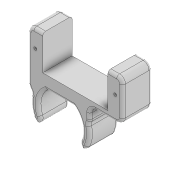
# Autodesk Inventor part: frame_3
Saved by Autodesk Inventor 2022 (Build 260153000, 153)
## iProperties
Created: 2023-05-17
Part Number: frame_3
Material: 일반
Document SubType Name: Modeling
Designer: HCI-TECH_KDK
Density: 1 g/cm^3
Appearance: 기본값
Author: HCI-TECH_KDK
Autodesk Inventor part; units mm, degrees
ref_plane "YZ Plane" through (0, 0, 0) normal (1, 0, 0) x (0, 1, 0)
ref_plane "XZ Plane" through (0, 0, 0) normal (0, 1, 0) x (-1, 0, 0)
ref_plane "XY Plane" through (0, 0, 0) normal (0, 0, 1) x (1, 0, 0)
sketch "스케치1" plane through (0, 0, 0) normal (0, 0, 1) x (1, 0, 0)
  line L0 (0, 0) -> (22.2, 0)
  line L1 (22.2, 0) -> (22.2, 11.8)
  line L2 (22.2, 11.8) -> (0, 11.8)
  line L3 (0, 11.8) -> (0, 0)
  circle A0 centre (6, 5.9) radius 1.877933
  line L4 (-9, 5.9) -> (21, 5.9)
  line L5 (21, 5.9) -> (21, -16.1)
  line L6 (21, -16.1) -> (-9, -16.1)
  line L7 (-9, -16.1) -> (-9, 5.9)
  line L8 (-24.543137, -4.6) -> (59.052201, -4.6) construction
  line L9 (-2, 5.9) -> (14, 5.9) construction
  line L10 (14, 5.9) -> (14, -16.1) construction
  line L11 (14, -16.1) -> (-2, -16.1) construction
  line L12 (-2, -16.1) -> (-2, 5.9) construction
  line L13 (-5, 11.8) -> (27.2, 11.8)
  line L14 (27.2, 11.8) -> (27.2, 0)
  line L15 (27.2, 0) -> (-5, 0)
  line L16 (-5, 0) -> (-5, 11.8)
  point P0 (6, 5.9)
  point P1 (6, 5.9)
  point P2 (0, 5.9)
  point P3 (11.1, 11.8)
  point P4 (11.1, 11.8)
  dimension "d0" = 22.2
  dimension "d1" = 11.8
  dimension "d2" = 6
  dimension "d3" = 22
  dimension "d4" = 30
  dimension "d5" = 11.5
  dimension "d6" = 16
  dimension "d10" = 32.2
  constraints: 34 end point, 8 parallel, 5 horizontal, 5 midpoint, 4 coincident, 4 perpendicular, 2 point on line, 1 centre point, 1 horizontal alignment
  measures "d0" distance of L1.end L2.end
  measures "d1" distance of L0.end L1.end
  measures "d2" distance from line of L3 A0.centre
  measures "d3" distance of L4.end L5.end
  measures "d4" distance of L5.end L6.end
  measures "d5" distance between parallel lines of L6 L8
  measures "d6" distance between parallel lines of L12 L10
  measures "d10" distance of L13.start L13.end
sketch "스케치2" plane through (0, 0, 0) normal (0, 0, 1) x (1, 0, 0)
  line L0 (-24.543137, -4.6) -> (59.052201, -4.6) construction
  line L1 (-2, -16.1) -> (-2, 5.9) construction
  line L2 (14, 5.9) -> (14, -16.1) construction
  line L3 (21, -16.1) -> (-9, -16.1)
  line L4 (-2, -4.6) -> (14, -4.6)
  line L5 (14, -4.6) -> (14, -16.1)
  line L6 (14, -16.1) -> (-2, -16.1)
  line L7 (-2, -16.1) -> (-2, -4.6)
  line L8 (-4, -18.1) -> (16, -18.1)
  line L9 (16, -18.1) -> (16, -2.6)
  line L10 (16, -2.6) -> (-4, -2.6)
  line L11 (-4, -2.6) -> (-4, -18.1)
  point P0 (0, 0)
  point P1 (-2, -16.1)
  dimension "d7" = 2
  dimension "d42" = 11.5
  dimension "d43" = 16
  constraints: 16 end point, 4 parallel, 2 perpendicular, 2 point on line, 1 horizontal, 3 other
  measures "d7" distance between parallel lines of L6 L8
  measures "d42" distance of L6.end L4.start
  measures "d43" distance between parallel lines of L2 L1
sketch "스케치2 outline for 돌출1" plane through (0, 0, 0) normal (0, 0, 1) x (1, 0, 0)
  line L0 (-4, -2.6) -> (-4, -18.1)
  line L1 (16, -2.6) -> (-4, -2.6)
  line L2 (-4, -18.1) -> (16, -18.1)
  line L3 (16, -18.1) -> (16, -2.6)
  line L4 (-2, -16.1) -> (-2, -4.6)
  line L5 (14, -16.1) -> (-2, -16.1)
  line L6 (14, -4.6) -> (14, -16.1)
  line L7 (-2, -4.6) -> (14, -4.6)
extrude "돌출1" add sketch "스케치2 outline for 돌출1" against normal blind 10
sketch "스케치3" plane through (0, 0, 0) normal (0, 0, 1) x (1, 0, 0)
  line L0 (0, 11.8) -> (0, 0)
  line L1 (-5, 11.8) -> (27.2, 11.8)
  line L2 (-5, 0) -> (-5, 11.8)
  line L3 (27.2, 0) -> (-5, 0)
  line L4 (27.2, 11.8) -> (27.2, 0)
  line L5 (22.2, 0) -> (22.2, 11.8)
  line L6 (27.2, 11.8) -> (22.2, 11.8)
  line L7 (27.2, 0) -> (27.2, -6.593642)
  line L8 (27.2, -6.593642) -> (16, -6.593642)
  line L9 (16, -2.6) -> (16, -18.1)
  line L10 (-9, -16.1) -> (-9, 5.9)
  line L11 (-4, -18.1) -> (-4, -2.6)
  line L12 (-4, -6.593642) -> (-9, -6.593642)
  line L13 (-9, 5.9) -> (0, 5.9)
  line L14 (21, 5.9) -> (21, -16.1)
  line L15 (0, 0) -> (22.2, 0)
  line L16 (16, -2.6) -> (-4, -2.6)
  line L17 (16, -18.1) -> (16, -2.6)
  point P0 (-5, 5.9)
  constraints: 10 end point, 3 point on line, 2 perpendicular, 1 collinear, 1 midpoint, 1 vertical
sketch "스케치3 outline for 돌출2" plane through (0, 0, 0) normal (0, 0, 1) x (1, 0, 0)
  line L0 (-4, -2.6) -> (16, -2.6)
  line L1 (-4, -6.593642) -> (-4, -2.6)
  line L2 (-9, -6.593642) -> (-4, -6.593642)
  line L3 (-9, 5.9) -> (-9, -6.593642)
  line L4 (-5, 5.9) -> (-9, 5.9)
  line L5 (-5, 11.8) -> (-5, 5.9)
  line L6 (0, 11.8) -> (-5, 11.8)
  line L7 (0, 0) -> (0, 11.8)
  line L8 (22.2, 0) -> (0, 0)
  line L9 (22.2, 11.8) -> (22.2, 0)
  line L10 (27.2, 11.8) -> (22.2, 11.8)
  line L11 (27.2, 0) -> (27.2, 11.8)
  line L12 (27.2, -6.593642) -> (27.2, 0)
  line L13 (16, -6.593642) -> (27.2, -6.593642)
  line L14 (16, -2.6) -> (16, -6.593642)
extrude "돌출2" add sketch "스케치3 outline for 돌출2" against normal blind 10
sketch "스케치4" plane through (0, 0, 0) normal (0, 0, 1) x (1, 0, 0)
  line L0 (-5, 11.8) -> (27.2, 11.8)
  line L1 (-5, 11.8) -> (-5, 5.9)
  line L2 (-5, 0) -> (-5, 11.8)
  line L3 (27.2, 0) -> (-5, 0)
  line L4 (27.2, -6.593642) -> (27.2, 11.8)
  line L5 (27.2, 11.8) -> (22.2, 11.8)
  line L6 (22.2, 11.8) -> (0, 11.8)
  line L7 (-5, 11.8) -> (0, 11.8)
  line L8 (0, 11.8) -> (0, 0)
  line L9 (0, 0) -> (-5, 0)
  line L10 (-5, 0) -> (-5, 11.8)
  line L11 (22.2, 11.8) -> (27.2, 11.8)
  line L12 (27.2, 11.8) -> (27.2, 0)
  line L13 (27.2, 0) -> (22.2, 0)
  line L14 (22.2, 0) -> (22.2, 11.8)
  circle A0 centre (-2.5, 5.9) radius 0.5
  circle A1 centre (24.7, 5.9) radius 0.5
  dimension "d13" = 1
  dimension "d14" = 1
  constraints: 16 end point, 4 parallel, 2 centre point, 2 horizontal, 2 perpendicular
  measures "d13" diameter of A0
  measures "d14" diameter of A1
sketch "스케치4 outline for 돌출3" plane through (0, 0, 0) normal (0, 0, 1) x (1, 0, 0)
  circle A0 centre (-2.5, 5.9) radius 0.5
  circle A1 centre (24.7, 5.9) radius 0.5
extrude "돌출3" cut sketch "스케치4 outline for 돌출3" against normal blind 6
sketch "스케치16" plane through (-9, 5.9, 0) normal (0, 1, 0) x (1, 0, 0)
  line L0 (4, 0) -> (0, 0) projected
  line L1 (4, 0) -> (4, 10) projected
  line L2 (0, 10) -> (4, 10) projected
  line L3 (0, 0) -> (0, 10) projected
  point P0 (9, 0)
sketch "스케치16 outline for 돌출11" plane through (-9, 5.9, 0) normal (0, 1, 0) x (1, 0, 0)
  line L0 (4, 0) -> (4, 10)
  line L1 (0, 0) -> (4, 0)
  line L2 (0, 10) -> (0, 0)
  line L3 (4, 10) -> (0, 10)
extrude "돌출11" cut sketch "스케치16 outline for 돌출11" against normal blind 32.25
sketch "스케치17" plane through (27.2, -6.593642, 0) normal (1, 0, 0) x (0, 0, -1)
  line L0 (0, 1.993642) -> (10, 1.993642)
  line L1 (0, 0) -> (10, 0)
  line L2 (10, 18.393642) -> (10, 0)
  line L3 (0, 0) -> (10, 0)
  line L4 (10, 0) -> (10, 4.419989)
  line L5 (10, 4.419989) -> (0, 4.419989)
  line L6 (0, 4.419989) -> (0, 0)
  point P0 (0, 6.593642)
  constraints: 8 end point, 2 parallel, 1 horizontal, 1 perpendicular, 1 point on line
sketch "스케치17 outline for 돌출12" plane through (27.2, -6.593642, 0) normal (1, 0, 0) x (0, 0, -1)
  line L0 (0, 4.419989) -> (0, 0)
  line L1 (10, 4.419989) -> (0, 4.419989)
  line L2 (10, 0) -> (10, 4.419989)
  line L3 (0, 0) -> (10, 0)
extrude "돌출12" cut sketch "스케치17 outline for 돌출12" against normal blind 11.2
sketch "Sketch18" plane through (0, 0, 0) normal (0, 0, 1) x (1, 0, 0)
  point P0 (0, 0)
sketch "Sketch20" plane through (0, 0, 0) normal (0, 0, 1) x (1, 0, 0)
  line L0 (16, -2.173653) -> (27.2, -2.173653)
  line L1 (27.2, -2.173653) -> (27.2, 11.8)
  line L2 (27.2, 11.8) -> (22.2, 11.8)
  line L3 (22.2, 11.8) -> (22.2, 0)
  line L4 (22.2, 0) -> (0, 0)
  line L5 (0, 0) -> (0, 11.8)
  line L6 (0, 11.8) -> (-5, 11.8)
  line L7 (-5, 11.8) -> (-5, -6.593642)
  line L8 (-5, -6.593642) -> (-4, -6.593642)
  line L9 (-4, -6.593642) -> (-4, -18.1)
  line L10 (-4, -18.1) -> (16, -18.1)
  line L11 (16, -18.1) -> (16, -2.173653)
  line L12 (-2, -16.1) -> (-2, -4.6)
  line L13 (-2, -4.6) -> (14, -4.6)
  line L14 (14, -4.6) -> (14, -16.1)
  line L15 (14, -16.1) -> (-2, -16.1)
  circle A0 centre (24.7, 5.9) radius 0.5
  circle A1 centre (-2.5, 5.9) radius 0.5
  line L16 (-4, -6.593642) -> (-5, -6.593642)
  line L17 (-5, -6.593642) -> (16, -6.593642)
  line L18 (16, -2.173653) -> (16, -18.1)
  point P0 (14, -6.593642)
  point P1 (-2, -6.593642)
  constraints: 2 end point, 1 perpendicular, 1 point on line
sketch "Sketch20 outline for Extrusion13" plane through (0, 0, 0) normal (0, 0, 1) x (1, 0, 0)
  line L0 (-4, -18.1) -> (16, -18.1)
  line L1 (-4, -6.593642) -> (-4, -18.1)
  line L2 (-2, -6.593642) -> (-4, -6.593642)
  line L3 (-2, -16.1) -> (-2, -6.593642)
  line L4 (14, -16.1) -> (-2, -16.1)
  line L5 (14, -6.593642) -> (14, -16.1)
  line L6 (16, -6.593642) -> (14, -6.593642)
  line L7 (16, -18.1) -> (16, -6.593642)
extrude "Extrusion13" cut sketch "Sketch20 outline for Extrusion13" against normal blind 10
sketch "Sketch21" plane through (0, 0, 0) normal (0, 0, 1) x (1, 0, 0)
  arc A0 (12.032825, -14.815463) -> (-0.254456, -14.815463) centre (5.889185, -10.513639) ccw
  arc A1 (14.111629, -16.271057) -> (-2.33326, -16.271057) centre (5.889185, -10.513639) ccw
  line L0 (5.889185, -10.513639) -> (-2.33326, -16.271057)
  line L1 (5.889185, -10.513639) -> (14.111629, -16.271057)
  line L2 (5.889185, -10.513639) -> (5.889185, 0)
  line L3 (0, 0) -> (22.2, 0)
  line L4 (-5, -6.593642) -> (-2, -6.593642)
  line L5 (-2, -6.593642) -> (-2, -4.6)
  line L6 (-2, -4.6) -> (14, -4.6)
  line L7 (14, -4.6) -> (14, -6.593642)
  line L8 (14, -6.593642) -> (16, -6.593642)
  line L9 (16, -6.593642) -> (16, -2.173653)
  line L10 (16, -2.173653) -> (27.2, -2.173653)
  line L11 (27.2, -2.173653) -> (27.2, 11.8)
  line L12 (27.2, 11.8) -> (22.2, 11.8)
  line L13 (22.2, 11.8) -> (22.2, 0)
  line L14 (22.2, 0) -> (0, 0)
  line L15 (0, 0) -> (0, 11.8)
  line L16 (0, 11.8) -> (-5, 11.8)
  line L17 (-5, 11.8) -> (-5, -6.593642)
  circle A2 centre (24.7, 5.9) radius 0.5
  circle A3 centre (-2.5, 5.9) radius 0.5
  dimension "d53" = 15
  dimension "d54" = 125
  dimension "d55" = 125
  constraints: 6 end point, 5 point on circle, 3 point on line, 2 centre point, 1 vertical
  measures "d53" diameter of A0
  measures "d54" angle of L2 L1
  measures "d55" angle of L2 L0
sketch "Sketch21 outline for Extrusion14" plane through (0, 0, 0) normal (0, 0, 1) x (1, 0, 0)
  line L0 (12.032825, -14.815463) -> (14.111629, -16.271057)
  arc A0 (-0.254456, -14.815463) -> (12.032825, -14.815463) centre (5.889185, -10.513639) cw
  line L1 (-2.33326, -16.271057) -> (-0.254456, -14.815463)
  arc A1 (14.111629, -16.271057) -> (-2.33326, -16.271057) centre (5.889185, -10.513639) ccw
extrude "Extrusion14" add sketch "Sketch21 outline for Extrusion14" against normal blind 10
fillet "Fillet6" radius 2 12 edges at (-0.2545, -14.8155, -5) (-2.3333, -16.2711, -5) (12.0328, -14.8155, -5) (14.1116, -16.2711, -5) (-5, -6.5936, -5) (-3.3515, -6.5936, -5) (16, -6.5936, -5) (15.1299, -6.5936, -5) (27.2, -2.1737, -5) (16, -2.1737, -5) (27.2, 11.8, -5) (-5, 11.8, -5)
fillet "Fillet7" radius 1 28 edges at (15.9509, -6.4993, -10) (16, -5.1162, -10) (15.6234, -7.5632, -10) (15.8765, -11.5186, -10) (-4.0707, -11.7616, -10) (-2.6214, -15.4603, -10) (27.2, 4.8132, -10) (23.7, 11.8, -10) (21.6, -2.1737, -10) (-5, 2.0731, -10) (-1.5, 11.8, -10) (15.9509, -6.4993, 0) (15.6234, -7.5632, 0) (-2.6214, -15.4603, 0) (23.7, 11.8, 0) (21.6, -2.1737, 0) (16, -5.1162, 0) (15.8765, -11.5186, 0) (-4.0707, -11.7616, 0) (27.2, 4.8132, 0) (-1.5, 11.8, 0) (-5, 2.0731, 0) (13.147, -8.6233, 0) (-1.3687, -8.6233, 0) (5.8892, -4.6, 0) (5.8892, -4.6, -10) (13.147, -8.6233, -10) (-1.3687, -8.6233, -10)
